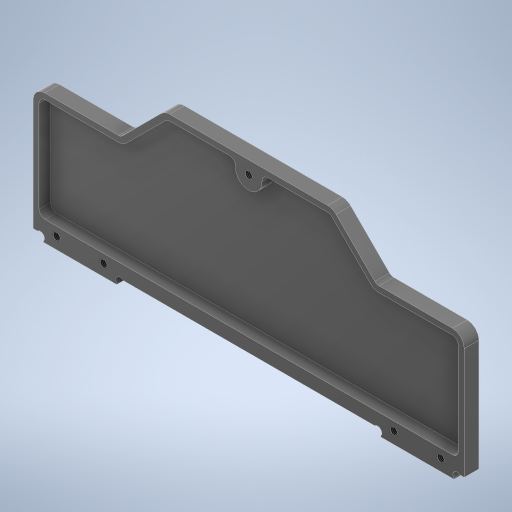
# Autodesk Inventor part: TorsoPelvisCoverFrame
Saved by Autodesk Inventor 2024.2 (Build 282272000, 272)
## iProperties
Created: 2024-01-11
Part Number: TorsoPelvisCoverFrame
Material: Acetal Resin, Black
Document SubType Name: Modeling
Designer: Masato Kubotera
Density: 1.425 g/cm^3
Appearance: Smooth - Black
Vendor: meviy
Mass: 17.716 g
Surface Area: 183.465 cm^2
Volume: 12.4323 cm^3
Author: Masato Kubotera
Autodesk Inventor part; units mm, degrees
ref_plane "YZ Plane" through (0, 0, 0) normal (1, 0, 0) x (0, 1, 0)
ref_plane "XZ Plane" through (0, 0, 0) normal (0, 1, 0) x (-1, 0, 0)
ref_plane "XY Plane" through (0, 0, 0) normal (0, 0, 1) x (1, 0, 0)
sketch "Sketch1" plane through (0, 0, 0) normal (1, 0, 0) x (0, 1, 0)
  line L0 (-73.5, -22.15) -> (73.5, -22.15) construction
  line L1 (73.5, 22.15) -> (-73.5, 22.15) construction
  line L2 (-73.5, 22.15) -> (-73.5, -22.15) construction
  line L3 (-73.5, -22.15) -> (73.5, 22.15) construction
  line L4 (73.5, -22.15) -> (-73.5, 22.15) construction
  line L5 (-73.5, 0) -> (73.5, 0) construction
  line L6 (0, 22.15) -> (0, -22.15) construction
  line L7 (49.5, -18.25) -> (65.5, -18.25) construction
  line L8 (45, -22.15) -> (45, -14.25) construction
  line L9 (45, -14.25) -> (70, -14.25) construction
  line L10 (70, -14.25) -> (70, -22.15) construction
  line L11 (57.5, -14.25) -> (57.5, -22.15) construction
  line L12 (-49.5, -18.25) -> (-65.5, -18.25) construction
  line L13 (-45, -22.15) -> (-45, -14.25) construction
  line L14 (-45, -14.25) -> (-70, -14.25) construction
  line L15 (-70, -14.25) -> (-70, -22.15) construction
  line L16 (-57.5, -14.25) -> (-57.5, -22.15) construction
  line L17 (-73.5, 17.15) -> (69, 17.15) construction
  line L18 (45, -22.15) -> (45, -19.85)
  line L19 (45, -19.85) -> (-45, -19.85)
  line L20 (-45, -19.85) -> (-45, -22.15)
  line L21 (-70, -20.35) -> (70, -20.35) construction
  line L22 (73.5, 22.15) -> (73.5, -22.15) construction
  line L23 (70, -22.15) -> (70, -19.85)
  line L24 (70, -19.85) -> (73.5, -19.85)
  line L25 (-70, -22.15) -> (-70, -19.85)
  line L26 (-70, -19.85) -> (-73.5, -19.85)
  line L27 (71.5, 20.15) -> (71.5, 8.9)
  line L28 (71.5, -15.25) -> (-71.5, -15.25)
  line L29 (71.5, 20.15) -> (-71.5, 20.15) construction
  circle A0 centre (49.5, -18.25) radius 3 construction
  line L30 (71.5, 20.15) -> (71.5, -15.25)
  line L31 (-71.5, 20.15) -> (-71.5, -15.25)
  line L32 (73.5, 22.15) -> (73.5, -19.85)
  line L33 (-73.5, 22.15) -> (-73.5, -19.85)
  line L34 (70, -22.15) -> (45, -22.15)
  line L35 (-45, -22.15) -> (-70, -22.15)
  arc A1 (72.1213, -19.85) -> (70, -21.9713) centre (71.0607, -20.9107) ccw
  arc A2 (45, -21.9713) -> (42.8787, -19.85) centre (43.9393, -20.9107) ccw
  arc A3 (-70, -21.9713) -> (-72.1213, -19.85) centre (-71.0607, -20.9107) ccw
  arc A4 (-42.8787, -19.85) -> (-45, -21.9713) centre (-43.9393, -20.9107) ccw
  line L36 (73.5, 23.15) -> (-73.5, 23.15) construction
  line L37 (43.5858, 22.15) -> (28.5858, 37.15)
  line L38 (28.5858, 37.15) -> (-28.5858, 37.15)
  line L39 (-28.5858, 37.15) -> (-43.5858, 22.15)
  line L40 (-44, 23.15) -> (-29, 38.15) construction
  line L41 (-29, 38.15) -> (29, 38.15) construction
  line L42 (29, 38.15) -> (44, 23.15) construction
  line L43 (42.7574, 20.15) -> (27.7574, 35.15)
  line L44 (27.7574, 35.15) -> (3.7417, 35.15)
  arc A5 (-3.7417, 35.15) -> (3.7417, 35.15) centre (0, 32.65) ccw
  line L45 (-42.7574, 20.15) -> (-27.7574, 35.15)
  line L46 (-27.7574, 35.15) -> (-3.7417, 35.15)
  line L47 (-71.5, 20.15) -> (-42.7574, 20.15)
  line L48 (-43.5858, 22.15) -> (-73.5, 22.15)
  line L49 (42.7574, 20.15) -> (71.5, 20.15)
  line L50 (73.5, 22.15) -> (43.5858, 22.15)
  point P0 (0, 0)
  point P1 (-73.5, -22.15)
  point P2 (-45, -22.15)
  point P3 (-45, -22.15)
  point P4 (-73.5, -19.85)
  point P5 (-70, -22.15)
  point P6 (-72.1213, -19.85)
  point P7 (-70, -21.9713)
  point P8 (-45, -21.9713)
  point P9 (-42.8787, -19.85)
  point P10 (42.8787, -19.85)
  point P11 (45, -21.9713)
  point P12 (-45, -19.85)
  point P13 (45, -19.85)
  point P14 (-70, -19.85)
  point P15 (-63.7555, -20)
  point P16 (-39.2445, -20)
  point P17 (39.2445, -20)
  point P18 (63.7555, -20)
  point P19 (71.5, 8.9)
  dimension "d0" = 147
  dimension "d2" = 16
  dimension "d3" = 3.9
  dimension "d4" = 25
  dimension "d5" = 7.9
  dimension "d18" = 5
  dimension "d35" = 2.1
  dimension "d36" = 0.5
  dimension "d38" = 115
  dimension "d47" = 2
  dimension "d50" = 6
  dimension "d53" = 2
  dimension "d56" = 1.5
  dimension "d57" = 42.5
  dimension "d59" = 1
  dimension "d60" = 14
  dimension "d63" = 45
  dimension "d64" = 15
  dimension "d65" = 1
  dimension "d66" = 1
  dimension "d67" = 88
  dimension "d68" = 43.5
  dimension "d69" = 4.5
  dimension "d70" = 2
  dimension "d71" = 2
  constraints: 102 end point, 31 symmetric about line, 21 point on line, 11 horizontal, 11 point on circle, 7 midpoint, 6 centre point, 6 coincident, 5 collinear, 5 vertical, 2 parallel, 2 tangent, 1 perpendicular, 5 other
  measures "d0" distance of L0.start L0.end
  measures "d2" distance of L7.start L7.end
  measures "d3" distance between parallel lines of L0 L7
  measures "d4" distance between parallel lines of L10 L8
  measures "d5" distance between parallel lines of L0 L9
  measures "d18" distance between parallel lines of L17 L1
  measures "d35" distance between parallel lines of L21 L7
  measures "d36" distance between parallel lines of L21 L19
  measures "d38" distance between parallel lines of L11 L16
  measures "d47" distance between parallel lines of L29 L1
  measures "d50" diameter of A0
  measures "d53" distance between parallel lines of L22 L30
  measures "d56" radius of A1
  measures "d57" distance between parallel lines of L21 L1
  measures "d59" distance between parallel lines of L1 L36
  measures "d60" distance between parallel lines of L36 L38
  measures "d63" angle of L36 L42
  measures "d64" distance between parallel lines of L36 L41
  measures "d65" distance between parallel lines of L38 L41
  measures "d66" distance between parallel lines of L37 L42
  measures "d67" distance of L42.end L40.start
  measures "d68" distance between parallel lines of L36 L21
  measures "d69" distance from line of point (0, 32.65) L38
  measures "d70" distance between parallel lines of L43 L37
  measures "d71" distance between parallel lines of L44 L38
extrude "Extrusion1" add sketch "Sketch1" against normal blind 5 contours L18 A2 L19 A4 L20 L35 L25 A3 L26 L33 L48 L39 L38 L37 L50 L32 L24 A1 L23 L34 | L27 L30 L28 L31 L47 L45 L46 A5 L44 L43 L49
extrude "Extrusion2" cut sketch "Sketch1" against normal blind 4 contours L27 L30 L28 L31 L47 L45 L46 A5 L44 L43 L49
hole "M3" at (0, 49.5, -18.25) at (0, 65.5, -18.25) at (0, -65.5, -18.25) at (0, -49.5, -18.25) at (0, 0, 32.65) direction (-1, 0, 0) diameter 2.459 end through all thread size "M3x0.5" class "6H" standard "ANSI Metric M Profile"
fillet "R2" radius 2 10 edges at (-2, 71.5, -15.25) (-2, -71.5, -15.25) (-2, -71.5, 20.15) (-2.5, -43.5858, 22.15) (-2.5, 43.5858, 22.15) (-2, -27.7574, 35.15) (-2, -3.7417, 35.15) (-2, 3.7417, 35.15) (-2, 27.7574, 35.15) (-2, 71.5, 20.15)
fillet "R4" radius 4 6 edges at (-2.5, 73.5, 22.15) (-2.5, -28.5858, 37.15) (-2.5, 28.5858, 37.15) (-2.5, -73.5, 22.15) (-2, -42.7574, 20.15) (-2, 42.7574, 20.15)
body "Solid1"
